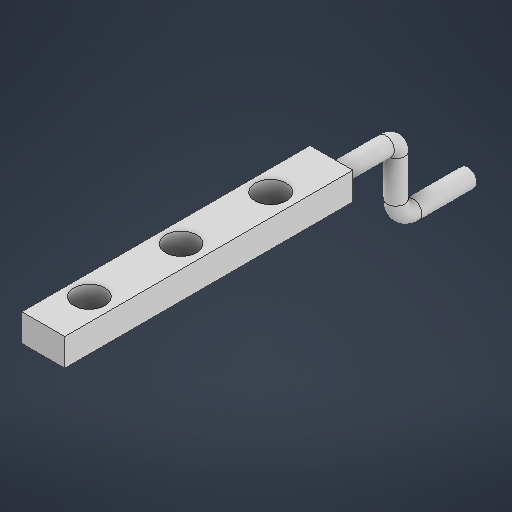
# Autodesk Inventor part: Slits
Saved by Autodesk Inventor 2026.1 (Build 301233020, 233B)
## iProperties
Created: 2025-11-11
Part Number: Slits
Material: Generic
Document SubType Name: Modeling
Designer: jacob
Density: 1 g/cm^3
Appearance: Default
Author: jacob
Autodesk Inventor part; units mm, degrees
ref_plane "YZ Plane" through (0, 0, 0) normal (1, 0, 0) x (0, 1, 0)
ref_plane "XZ Plane" through (0, 0, 0) normal (0, 1, 0) x (-1, 0, 0)
ref_plane "XY Plane" through (0, 0, 0) normal (0, 0, 1) x (1, 0, 0)
sketch "Sketch1" plane through (0, 0, 0) normal (0, 1, 0) x (-1, 0, 0)
  line L0 (3.0162, -25.0369) -> (-3.2338, -25.0369)
  line L1 (3.0162, -25.0369) -> (3.0162, 16.9631)
  line L2 (3.0162, 16.9631) -> (-3.2338, 16.9631)
  line L3 (-3.2338, 16.9631) -> (-3.2338, -25.0369)
  point P0 (0, 0)
  dimension "d1" = 6.25
  dimension "d3" = 42
  constraints: 8 end point, 2 perpendicular, 1 vertical
  measures "d1" distance of L0.start L0.end
  measures "d3" distance of L0.start L1.end
extrude "Extrusion1" add sketch "Sketch1" along normal blind 4
sketch "Sketch10" plane through (3.2338, 0, -25.0369) normal (0, 0, -1) x (-1, 0, 0)
  circle A0 centre (3.2338, 1.4878) radius 1.2786
  point P0 (3.2338, 0)
  constraints: 1 centre point
sketch "Sketch12" plane through (0, 0, 0) normal (1, 0, 0) x (0, 1, 0)
  line L0 (0, -25.0369) -> (4, -25.0369) projected
  line L1 (2, -25.0369) -> (2, -33.0369)
  line L2 (0, -35.0369) -> (-6, -35.0369)
  line L3 (-8, -37.0369) -> (-8, -45.0369)
  arc A0 (0, -35.0369) -> (2, -33.0369) centre (0, -33.0369) ccw
  arc A1 (-6, -35.0369) -> (-8, -37.0369) centre (-6, -37.0369) ccw
  point P0 (0, 0)
  point P1 (2, -35.0369)
  point P2 (-8, -35.0369)
  dimension "d15" = 10
  dimension "d16" = 10
  dimension "d17" = 10
  dimension "d18" = 2
  constraints: 6 end point, 4 point on circle, 4 point on line, 4 tangent, 2 centre point, 2 perpendicular, 1 equal radius, 1 midpoint, 1 vertical
  measures "d15" distance of L1.start point (2, -35.037)
  measures "d16" distance of point (2, -35.037) point (-8, -35.037)
  measures "d17" distance of point (-8, -35.037) L3.end
  measures "d18" radius of A0
sweep "Sweep1" add profiles "Sketch10" path "Sketch12" path curves L1 A0 L2 A1 L3
sketch "Sketch14" plane through (0, 4, 0) normal (0, 1, 0) x (1, 0, 0)
  circle A0 centre (0, 3.2271) radius 2.25
  circle A1 centre (0, 16.2844) radius 2.25
  circle A2 centre (0, -10.1533) radius 2.25
  point P0 (0, 0)
  dimension "d29" = 4.5
  dimension "d30" = 4.5
  dimension "d31" = 4.5
  constraints: 3 centre point
  measures "d29" diameter of A0
  measures "d30" diameter of A1
  measures "d31" diameter of A2
extrude "Extrusion5" cut sketch "Sketch14" against normal blind 3.2
body "Solid1"
